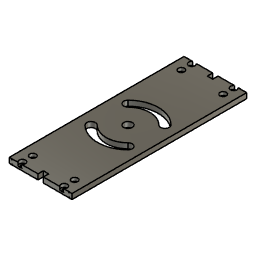
FS80+UL Pivot Base v9 (Autodesk Fusion 360 design; units mm, degrees)
Autodesk Fusion 360 part; units mm, degrees
sketch "Schizzo5" plane through (0, 0, 0) normal (0, 0, 1) x (1, 0, 0)
  line L0 (75.1728, 108.9816) -> (75.1728, -58.2184)
  circle A0 centre (85.1728, -55.7184) radius 1.5
  circle A1 centre (125.1728, 106.4816) radius 3
  line L1 (75.1728, 25.3816) -> (135.1728, 25.3816) construction
  circle A2 centre (85.1728, 106.4816) radius 3
  line L2 (105.1728, 25.3816) -> (122.8504, 7.7039) construction
  circle A3 centre (85.1728, 106.4816) radius 1.5
  line L3 (135.1728, 108.9816) -> (75.1728, 108.9816)
  circle A4 centre (125.1728, 106.4816) radius 1.5
  line L4 (105.1728, 25.3816) -> (87.4951, 43.0593) construction
  line L5 (105.1728, 25.3816) -> (105.1728, 1.3102) construction
  circle A5 centre (105.1728, 25.3816) radius 4.1
  line L6 (135.1728, -58.2184) -> (135.1728, 108.9816)
  line L7 (85.1728, 108.9816) -> (85.1728, -58.2184) construction
  circle A6 centre (85.1728, -55.7184) radius 3
  circle A7 centre (125.1728, -55.7184) radius 1.5
  line L8 (105.1728, 25.3816) -> (122.8504, 43.0593) construction
  line L9 (75.1728, -58.2184) -> (135.1728, -58.2184)
  circle A8 centre (125.1728, -55.7184) radius 3
  line L10 (75.1728, -55.7184) -> (135.1728, -55.7184) construction
  line L11 (105.1728, 25.3816) -> (87.4951, 7.7039) construction
  line L12 (105.1728, 108.9816) -> (105.1728, -58.2184) construction
  line L13 (105.1728, 25.3816) -> (105.1728, 56.9762) construction
  line L14 (105.1728, 25.3816) -> (105.1728, 56.9762) construction
  line L15 (105.1728, 25.3816) -> (105.1728, 1.3102) construction
  line L16 (75.1728, -45.7184) -> (135.1728, -45.7184) construction
  circle A9 centre (85.1728, -45.7184) radius 1.5
  circle A10 centre (85.1728, -45.7184) radius 3
  circle A11 centre (125.1728, -45.7184) radius 3
  circle A12 centre (125.1728, -45.7184) radius 1.5
  circle A13 centre (85.1728, 96.4816) radius 3
  circle A14 centre (85.1728, 96.4816) radius 1.5
  circle A15 centre (125.1728, 96.4816) radius 3
  circle A16 centre (125.1728, 96.4816) radius 1.5
  line L17 (107.7228, -58.2184) -> (102.6228, -58.2184)
  line L18 (102.6228, -58.2184) -> (102.6228, -53.1184)
  line L19 (102.6228, -53.1184) -> (107.7228, -53.1184)
  line L20 (107.7228, -53.1184) -> (107.7228, -58.2184)
  line L21 (107.7228, -58.2184) -> (102.6228, -53.1184) construction
  line L22 (102.6228, -58.2184) -> (107.7228, -53.1184) construction
  line L23 (102.6228, 103.8816) -> (107.7228, 103.8816)
  line L24 (102.6228, 108.9816) -> (102.6228, 103.8816)
  line L25 (107.7228, 103.8816) -> (107.7228, 108.9816)
  circle A17 centre (105.1728, 25.3816) radius 25 construction
  circle A18 centre (87.4951, 43.0593) radius 4.1
  circle A19 centre (122.8504, 7.7039) radius 4.1
  circle A20 centre (122.8504, 43.0593) radius 4.1
  circle A21 centre (87.4951, 7.7039) radius 4.1
  line L26 (87.4951, 7.7039) -> (84.596, 4.8048) construction
  line L27 (122.8504, 7.7039) -> (125.7496, 4.8048) construction
  arc A22 (84.596, 4.8048) -> (125.7496, 4.8048) centre (105.1728, 25.3816) ccw
  arc A23 (90.3942, 10.6031) -> (119.9513, 10.6031) centre (105.1728, 25.3816) ccw
  line L28 (87.4951, 43.0593) -> (84.596, 45.9584) construction
  line L29 (122.8504, 43.0593) -> (125.7496, 45.9584) construction
  arc A24 (125.7496, 45.9584) -> (84.596, 45.9584) centre (105.1728, 25.3816) ccw
  arc A25 (119.9513, 40.1601) -> (90.3942, 40.1601) centre (105.1728, 25.3816) ccw
  point P0 (105.1728, -55.6684)
  point P1 (105.1728, 25.3816)
  point P2 (87.4951, 7.7039)
  point P3 (122.8504, 7.7039)
  point P4 (122.8504, 43.0593)
  point P5 (87.4951, 43.0593)
  point P6 (84.596, 4.8048)
  point P7 (125.7496, 4.8048)
  point P8 (90.3942, 10.6031)
  point P9 (119.9513, 10.6031)
  point P10 (84.596, 45.9584)
  point P11 (125.7496, 45.9584)
  dimension "d221" = 60
  dimension "d222" = 167.2
  dimension "d223" = 2.5
  dimension "d224" = 20
  dimension "d225" = 3
  dimension "d226" = 6
  dimension "d229" = 8.2
  dimension "d350" = 3
  dimension "d351" = 6
  dimension "d354" = 10
  dimension "d355" = 5.1
  dimension "d356" = 5.1
  dimension "d361" = 50
  dimension "d362" = 8.2
  dimension "d363" = 8.2
  dimension "d364" = 45
  dimension "d365" = 45
  dimension "d366" = 45
  dimension "d367" = 45
  constraint horizontal L9
  constraint vertical L6
  constraint horizontal L3
  constraint vertical L0
  constraint midpoint L12.start L3
  constraint midpoint L12.end L9
  constraint coincident L10.end L6
  constraint perpendicular L6 L10
  constraint midpoint L1.start L0
  constraint midpoint L1.end L6
  constraint coincident L7.start L3
  constraint coincident L7.end L9
  constraint perpendicular L7 L9
  constraint coincident A0.centre L10
  constraint coincident A0.centre L7
  constraint concentric A0 A6
  constraint symmetric A0 A7 L12
  constraint symmetric A6 A8 L12
  constraint symmetric A0 L1 A3
  constraint symmetric L1 A2 A6
  constraint symmetric L1 A4 A7
  constraint symmetric A1 L1 A8
  constraint midpoint P1 L1
  constraint coincident L5.end L12
  constraint coincident P1 L2.start
  constraint coincident L13.end L12
  constraint coincident L10.start L0
  constraint coincident L0 L16.start
  constraint coincident L6 L16.end
  constraint perpendicular L6 L16
  constraint coincident L16 A9.centre
  constraint coincident L7 A9.centre
  constraint concentric A9 A10
  constraint symmetric L12 A9 A12
  constraint symmetric L12 A10 A11
  constraint collinear L8 L11
  constraint collinear L2 L4
  constraint symmetric L1 A9 A14
  constraint symmetric L1 A10 A13
  constraint symmetric L1 A11 A15
  constraint symmetric L1 A12 A16
  constraint horizontal L17
  constraint perpendicular L17 L18
  constraint parallel L17 L19
  constraint parallel L18 L20
  constraint coincident L21 P0
  constraint coincident L22 P0
  constraint coincident L12 P0
  constraint collinear L9 L17
  constraint symmetric L1 L17.start L25.end
  constraint symmetric L1 L17.end L24.start
  constraint symmetric L1 L18.end L23.start
  constraint symmetric L1 L19.end L23.end
  constraint concentric A5 A17
  constraint coincident P2 A17
  constraint coincident P3 A17
  constraint coincident P4 A17
  constraint coincident P5 A17
  constraint coincident P2 L11.end
  constraint coincident P3 L2.end
  constraint coincident P4 L8.end
  constraint coincident P5 L4.end
  constraint symmetric L8 A18 A19
  constraint symmetric L2 A20 A21
  constraint coincident A21 P6
  constraint coincident A19 P7
  constraint collinear L11 L26
  constraint collinear L2 L27
  constraint coincident P6 L26.end
  constraint coincident P7 L27.end
  constraint coincident L11 P8
  constraint coincident A21 P8
  constraint coincident A19 P9
  constraint coincident L2 P9
  constraint coincident P9 A23.end
  constraint coincident P8 A23.start
  constraint coincident A18 P10
  constraint coincident A20 P11
  constraint collinear L4 L28
  constraint collinear L8 L29
  constraint coincident P10 L28.end
  constraint coincident P11 L29.end
  constraint coincident A20 A25.start
  constraint coincident A18 A25.end
  constraint coincident L4 A25.end
  measures "d221" distance of L0.end L6.start
  measures "d222" distance of L0.end L0.start
  measures "d223" distance of L9 L10
  measures "d224" distance of L7 L12
  measures "d225" diameter of A0
  measures "d226" diameter of A6
  measures "d229" diameter of A5
  measures "d350" diameter of A9
  measures "d351" diameter of A10
  measures "d354" distance of L10 L16
  measures "d355" distance of L18.end L19.end
  measures "d356" distance of L17.end L18.end
  measures "d361" diameter of A17
  measures "d362" diameter of A18
  measures "d363" diameter of A20
  measures "d364" angle of L4 L12
  measures "d365" angle of L8 L12
  measures "d366" angle of L11 L12
  measures "d367" angle of L2 L12
extrude "Estrusione24" add sketch "Schizzo5" along normal blind 5 contours L0 A1 A2 L3 L6 A6 L9 A8 L18 L19 L20 L23 L24 L25
extrude "Estrusione25" add sketch "Schizzo5" along normal blind 1.8 contours A2 L3 | A6 L9 | A1 L3 | L9 A8 | A10 | A11 | A13 | A15 picked at (85.2101, 108.6469) picked at (85.2101, -57.8837) picked at (125.2101, 108.6469) picked at (125.2101, -57.8837)
sketch "Schizzo17" plane through (0, -58.2184, 0) normal (0, -1, 0) x (1, 0, 0)
  line L0 (75.1728, 0) -> (102.6228, 0)
  line L1 (102.6228, 0) -> (102.6228, 5)
  line L2 (102.6228, 5) -> (86.8311, 5)
  line L3 (86.8311, 5) -> (86.8311, 1.8)
  line L4 (86.8311, 1.8) -> (83.5144, 1.8)
  line L5 (83.5144, 1.8) -> (83.5144, 5)
  line L6 (83.5144, 5) -> (75.1728, 5)
  line L7 (75.1728, 5) -> (75.1728, 0)
  line L8 (75.1728, 5) -> (135.1728, 5) construction
  line L9 (135.1728, 5) -> (135.1728, 0) construction
  line L10 (135.1728, 0) -> (75.1728, 0) construction
  line L11 (75.1728, 0) -> (75.1728, 5) construction
  line L12 (107.7228, 0) -> (135.1728, 0) construction
  line L13 (107.7228, 5) -> (123.5144, 5) construction
  line L14 (135.1728, 0) -> (135.1728, 5) construction
  line L15 (75.1728, 2.5) -> (135.1728, 2.5) construction
  line L16 (77.9024, 5) -> (77.9024, 0) construction
  circle A0 centre (77.9024, 4.5) radius 0.4
  circle A1 centre (77.9024, 0.5) radius 0.4
  line L17 (105.1728, 5) -> (105.1728, 0) construction
  line L18 (132.4431, 5) -> (132.4431, 0) construction
  circle A2 centre (132.4431, 0.5) radius 0.4
  circle A3 centre (132.4431, 4.5) radius 0.4
  point P0 (132.4431, 4.5)
  point P1 (132.4431, 0.5)
  point P2 (132.4431, 4.5)
  dimension "d357" = 0.8
  dimension "d358" = 4
  constraint horizontal L8
  constraint vertical L9
  constraint horizontal L10
  constraint vertical L11
  constraint collinear L10 L12
  constraint collinear L8 L13
  constraint collinear L7 L11
  constraint collinear L9 L14
  constraint midpoint L7 L15.start
  constraint midpoint L9 L15.end
  constraint coincident L8 L16.start
  constraint coincident L10 L16.end
  constraint coincident L16 A0.centre
  constraint symmetric L15 A0 A1
  constraint midpoint L8 L17.start
  constraint midpoint L10 L17.end
  constraint symmetric L16.start L17 L18.start
  constraint symmetric L16.end L17 L18.end
  constraint symmetric A0.centre L17 P2
  constraint symmetric A1.centre L17 P1
  constraint symmetric A1 L17 A2
  constraint symmetric A0 L17 A3
  measures "d357" diameter of A0
  measures "d358" distance of A0.centre A1.centre
extrude "Estrusione29" cut sketch "Schizzo17" against normal blind 180 contours A0 | A1 | A2 | A3
equation "d225 = d227"
equation "d226 = d228"
equation "d227 = 3.00 mm"
equation "d228 = 6.00 mm"
equation "d350 = d227"
equation "d351 = d228"
equation "d362 = d229"
equation "d363 = d362"
named bodies: "Base"
